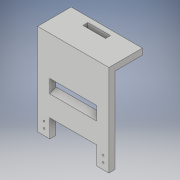
# Autodesk Inventor part: 0724
Saved by Autodesk Inventor 2019 (Build 230136000, 136)
## iProperties
Created: 2018-07-24
Part Number: 0724
Material: 一般
Document SubType Name: Modeling
Designer: j13tw
Density: 1 g/cm^3
Appearance: 預設
Author: j13tw
Autodesk Inventor part; units mm, degrees
ref_plane "YZ Plane" through (0, 0, 0) normal (1, 0, 0) x (0, 1, 0)
ref_plane "XZ Plane" through (0, 0, 0) normal (0, 1, 0) x (-1, 0, 0)
ref_plane "XY Plane" through (0, 0, 0) normal (0, 0, 1) x (1, 0, 0)
sketch "草圖1" plane through (0, 0, 0) normal (0, 0, 1) x (1, 0, 0)
  line L0 (-56.5, 30) -> (-36.5, 30)
  line L1 (-36.5, 30) -> (-36.5, 0)
  line L2 (-36.5, 0) -> (-56.5, 0)
  line L3 (-56.5, 0) -> (-56.5, 30)
  point P0 (0, 0)
  dimension "d0" = 30
  dimension "d1" = 20
  dimension "d2" = 36.5
  constraints: 8 end point, 2 parallel, 1 horizontal, 1 perpendicular
  measures "d0" distance of L0.end L1.end
  measures "d1" distance of L0.start L0.end
  measures "d2" distance of point (0, 0) L1.end
extrude "擠出1" add sketch "草圖1" along normal blind 5
sketch "草圖4" plane through (-56.5, 30, 0) normal (0, 1, 0) x (1, 0, 0)
  line L0 (0, 0) -> (58.5, 0)
  line L1 (58.5, 0) -> (58.5, -5)
  line L2 (58.5, -5) -> (0, -5)
  line L3 (0, -5) -> (0, 0)
  line L4 (20, -5) -> (0, -5) projected
  point P0 (56.5, 0)
  point P1 (18.5, -5)
  point P2 (3, -5)
  dimension "d20" = 5
  dimension "d21" = 0
  dimension "d87" = 58.5
  constraints: 8 end point, 2 parallel, 1 horizontal, 1 perpendicular
  measures "d20" distance of L2.end L0.start
  measures "d21" distance between parallel lines of L4 L2
  measures "d87" distance of L1.end L2.end
extrude "擠出4" add sketch "草圖4" along normal blind 120
mirror "鏡射1" about plane through (2, 30, 5) normal (1, 0, 0)
sketch "草圖5" plane through (0, 0, 0) normal (0, 0, -1) x (-1, 0, 0)
  line L0 (56.5, 150) -> (-60.5, 150) projected
  line L1 (-60.5, 150) -> (56.5, 150)
  line L2 (56.5, 150) -> (56.5, 140)
  line L3 (56.5, 140) -> (-60.5, 140)
  line L4 (-60.5, 140) -> (-60.5, 150)
  point P0 (0, 0)
  dimension "d24" = 10
  dimension "d25" = 117
  constraints: 8 end point, 2 parallel, 1 horizontal, 1 perpendicular
  measures "d24" distance of L1.end L2.end
  measures "d25" distance of L2.end L3.end
extrude "擠出5" add sketch "草圖5" along normal blind 50
sketch "草圖6" plane through (-56.5, 150, 0) normal (0, 1, 0) x (1, 0, 0)
  line L0 (36, 33.5) -> (73, 33.5)
  line L1 (73, 33.5) -> (73, 41.5)
  line L2 (73, 41.5) -> (36, 41.5)
  line L3 (36, 41.5) -> (36, 33.5)
  line L4 (0, -5) -> (117, -5) projected
  point P0 (56.5, 0)
  dimension "d28" = 37
  dimension "d29" = 16.5
  dimension "d30" = 8
  dimension "d31" = 38.5
  constraints: 8 end point, 2 parallel, 1 horizontal, 1 perpendicular
  measures "d28" distance of L1.end L2.end
  measures "d29" distance from line of L1 point (56.5, 0)
  measures "d30" distance of L0.end L1.end
  measures "d31" distance between parallel lines of L4 L0
extrude "擠出6" cut sketch "草圖6" against normal up to next
sketch "草圖7" plane through (0, 0, 0) normal (0, 0, -1) x (-1, 0, 0)
  line L0 (56.5, 140) -> (-60.5, 140) projected
  line L1 (-60.5, 0) -> (-60.5, 140) projected
  line L2 (-40.5, 0) -> (-60.5, 0) projected
  line L3 (-40.5, 30) -> (-40.5, 0) projected
  line L4 (36.5, 30) -> (-40.5, 30) projected
  line L5 (36.5, 30) -> (36.5, 0) projected
  line L6 (36.5, 0) -> (56.5, 0) projected
  line L7 (56.5, 0) -> (56.5, 140) projected
  point P0 (0, 0)
extrude "擠出7" add sketch "草圖7" along normal blind 5
sketch "草圖11" plane through (0, 0, 5) normal (0, 0, 1) x (1, 0, 0)
  line L0 (-36.5, 86) -> (40.5, 86)
  line L1 (40.5, 86) -> (40.5, 64)
  line L2 (40.5, 64) -> (-36.5, 64)
  line L3 (-36.5, 64) -> (-36.5, 86)
  line L4 (40.5, 0) -> (40.5, 30) projected
  line L5 (-36.5, 0) -> (-36.5, 30) projected
  line L6 (40.5, 30) -> (-36.5, 30) projected
  line L7 (-56.5, 150) -> (60.5, 150) projected
  point P0 (0, 0)
  dimension "d64" = 0
  dimension "d65" = 0
  dimension "d66" = 34
  dimension "d67" = 64
  constraints: 8 end point, 2 parallel, 1 horizontal, 1 perpendicular
  measures "d64" distance between parallel lines of L4 L1
  measures "d65" distance between parallel lines of L5 L3
  measures "d66" distance between parallel lines of L6 L2
  measures "d67" distance between parallel lines of L7 L0
sketch "草圖12" plane through (0, 0, -5) normal (0, 0, -1) x (-1, 0, 0)
  line L0 (-40.5, 90) -> (36.5, 90)
  line L1 (36.5, 90) -> (36.5, 69)
  line L2 (36.5, 69) -> (-40.5, 69)
  line L3 (-40.5, 69) -> (-40.5, 90)
  line L4 (36.5, 30) -> (36.5, 0) projected
  line L5 (-40.5, 0) -> (-40.5, 30) projected
  line L6 (-60.5, 140) -> (56.5, 140) projected
  line L7 (-40.5, 30) -> (36.5, 30) projected
  point P0 (0, 0)
  dimension "d68" = 0
  dimension "d69" = 0
  dimension "d70" = 50
  dimension "d71" = 39
  constraints: 8 end point, 2 parallel, 1 horizontal, 1 perpendicular
  measures "d68" distance between parallel lines of L4 L1
  measures "d69" distance between parallel lines of L5 L3
  measures "d70" distance between parallel lines of L6 L0
  measures "d71" distance between parallel lines of L7 L2
loft "斷面混成2" cut profiles "草圖11", "草圖12"
sketch "草圖13" plane through (0, 0, 5) normal (0, 0, 1) x (1, 0, 0)
  circle A0 centre (-45.75, 10.35) radius 1.25
  line L0 (-56.5, 0) -> (-56.5, 150) projected
  line L1 (-56.5, 0) -> (-36.5, 0) projected
  circle A1 centre (-45.75, 20.7) radius 1.25
  circle A2 centre (51.25, 10.35) radius 1.25
  circle A3 centre (51.25, 20.7) radius 1.25
  line L2 (40.5, 0) -> (40.5, 30) projected
  line L3 (60.5, 0) -> (40.5, 0) projected
  point P0 (0, 0)
  dimension "d76" = 2.5
  dimension "d77" = 10.75
  dimension "d78" = 10.35
  dimension "d79" = 10.35
  dimension "d80" = 10.75
  dimension "d81" = 10.75
  dimension "d82" = 10.75
  dimension "d83" = 10.35
  dimension "d84" = 10.35
  constraints: 4 centre point, 3 equal radius
  measures "d76" diameter of A0
  measures "d77" distance from line of L0 A0.centre
  measures "d78" distance from line of L1 A0.centre
  measures "d79" distance of A0.centre A1.centre
  measures "d80" distance from line of L0 A1.centre
  measures "d81" distance from line of L2 A2.centre
  measures "d82" distance from line of L2 A3.centre
  measures "d83" distance from line of L3 A2.centre
  measures "d84" distance of A2.centre A3.centre
extrude "擠出10" cut sketch "草圖13" against normal up to surface (10 mm away)
